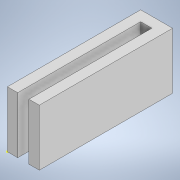
# Autodesk Inventor part: CouplerFAA
Saved by Autodesk Inventor 2020.1 (Build 241239000, 239)
## iProperties
Created: 2019-11-19
Part Number: CouplerFAA
Material: Generic
Document SubType Name: Modeling
Designer: super
Density: 1 g/cm^3
Appearance: Default
Author: super
Autodesk Inventor part; units mm, degrees
ref_plane "YZ Plane" through (0, 0, 0) normal (1, 0, 0) x (0, 1, 0)
ref_plane "XZ Plane" through (0, 0, 0) normal (0, 1, 0) x (-1, 0, 0)
ref_plane "XY Plane" through (0, 0, 0) normal (0, 0, 1) x (1, 0, 0)
sketch "Sketch1" plane through (0, 0, 0) normal (0, 1, 0) x (-1, 0, 0)
  line L0 (0, 0) -> (0, -65.5)
  line L1 (0, -65.5) -> (6, -65.5)
  line L2 (6, -65.5) -> (6, 0)
  line L3 (6, 0) -> (11.5, 0)
  line L4 (11.5, 0) -> (11.5, -71)
  line L5 (11.5, -71) -> (-5.5, -71)
  line L6 (-5.5, -71) -> (-5.5, 0)
  line L7 (-5.5, 0) -> (0, 0)
  dimension "d0" = 65.5
  dimension "d1" = 6
  dimension "d2" = 5.5
  dimension "d3" = 71
  dimension "d4" = 17
  constraints: 16 end point, 7 perpendicular, 1 point on line, 1 vertical
  measures "d0" distance of L0.start L0.end
  measures "d1" distance of L0.end L1.end
  measures "d2" distance of L2.end L3.end
  measures "d3" distance of L3.end L4.end
  measures "d4" distance of L4.end L5.end
extrude "Extrusion1" add sketch "Sketch1" along normal blind 30
sketch "Sketch2" plane through (-11.5, 0, -71) normal (-1, 0, 0) x (0, 0, 1)
  point P0 (71, 0)
body "Solid1"
